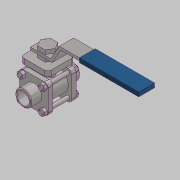
# Autodesk Inventor part: MANUAL BUTT WELD BALL VALVE DN15 304L
Saved by Autodesk Inventor 2017 (Build 210142000, 142)
## iProperties
Category: Plant Design Equipment
Company: Pocket Brewery Belgium
Created: 2017-11-25
Part Number: MANUAL BUTT WELD BALL VALVE DN15 304L
Material: 304L
Document SubType Name: Modeling
Designer: Demarec
Density: 8 g/cm^3
Appearance: Semi-Polished(1)
Description: BELVEN BV3
Author: Marc Crauwels
Title: Valves
Comments: This Valve is generated with the Pocket Brewery Valve App. This software is part of the Pocket Brewery Design Suite.
Autodesk Inventor part; units mm, degrees
ref_plane "YZ Plane" through (0, 0, 0) normal (1, 0, 0) x (0, 1, 0)
ref_plane "XZ Plane" through (0, 0, 0) normal (0, 1, 0) x (-1, 0, 0)
sketch "Sketch3" plane through (0, 0, 0) normal (0, 1, 0) x (-1, 0, 0)
  line L0 (-4.0756, 9.8393) -> (4.0756, 9.8393)
  line L1 (4.0756, 9.8393) -> (9.8393, 4.0756)
  line L2 (9.8393, 4.0756) -> (9.8393, -4.0756)
  line L3 (9.8393, -4.0756) -> (4.0756, -9.8393)
  line L4 (4.0756, -9.8393) -> (-4.0756, -9.8393)
  line L5 (-4.0756, -9.8393) -> (-9.8393, -4.0756)
  line L6 (-9.8393, -4.0756) -> (-9.8393, 4.0756)
  line L7 (-9.8393, 4.0756) -> (-4.0756, 9.8393)
  circle A0 centre (0, 0) radius 10.65
  line L8 (14.25, -19) -> (-14.25, -19)
  line L9 (-19, -14.25) -> (-19, 14.25)
  line L10 (-14.25, 19) -> (14.25, 19)
  line L11 (19, 14.25) -> (19, -14.25)
  line L12 (19, -19) -> (-19, 19) construction
  line L13 (-19, -19) -> (19, 19) construction
  circle A1 centre (0, 0) radius 9.8393
  arc A2 (19, 14.25) -> (14.25, 19) centre (14.25, 14.25) ccw
  arc A3 (-14.25, 19) -> (-19, 14.25) centre (-14.25, 14.25) ccw
  arc A4 (-19, -14.25) -> (-14.25, -19) centre (-14.25, -14.25) ccw
  arc A5 (14.25, -19) -> (19, -14.25) centre (14.25, -14.25) ccw
  circle A6 centre (0, 0) radius 8
  circle A7 centre (14.25, 14.25) radius 2.5
  circle A8 centre (0, 0) radius 14.65
  dimension "oSW" = 21.3
  dimension "oFlangeW" = 38
  dimension "d2" = 4.75
  dimension "oIntDia" = 16
  dimension "oMbolt" = 5
  dimension "d16" = 4
  constraints: 28 end point, 9 tangent, 8 centre point, 8 point on circle, 8 point on line, 5 coincident, 3 equal radius, 2 horizontal, 2 midpoint, 2 parallel, 2 perpendicular, 20 other
  measures "oFlangeW" distance of L12.start L13.start
  measures "d2" radius of A2
  measures "oIntDia" diameter of A6
  measures "oMbolt" diameter of A7
extrude "Extrusion1" add sketch "Sketch3" along normal mid plane 65 contours A0 L0 | L0 A1 L7 | L7 A0 | L0 L1 A1 | A1 | A1 L6 L7 | A0 L1 | L6 A0 | L1 L2 A1 | A1 L5 L6 | A0 L2 | L5 A0 | L2 L3 A1 | A1 L4 L5 | L4 A0 | A0 L3 | L3 L4 A1
extrude "Extrusion2" add sketch "Sketch3" along normal mid plane 37 contours A0 L0 | L7 A0 | A0 L1 | L6 A0 | A0 L2 | L5 A0 | L4 A0 | A0 L3 | L8 A4 L9 A3 L10 A2 L11 A5 | A7 | A8
extrude "Extrusion3" cut sketch "Sketch3" along normal mid plane 25 contours L8 A4 L9 A3 L10 A2 L11 A5 | A7
extrude "Extrusion4" add sketch "Sketch3" along normal mid plane 48 contours A7
sketch "Sketch4" plane through (0, -18.5, 0) normal (0, -1, 0) x (1, 0, 0)
  circle A0 centre (-14.25, 14.25) radius 2.5 projected
  line L0 (-12.0849, 10.5) -> (-16.4151, 10.5)
  line L1 (-16.4151, 10.5) -> (-18.5801, 14.25)
  line L2 (-18.5801, 14.25) -> (-16.4151, 18)
  line L3 (-16.4151, 18) -> (-12.0849, 18)
  line L4 (-12.0849, 18) -> (-9.9199, 14.25)
  line L5 (-9.9199, 14.25) -> (-12.0849, 10.5)
  point P0 (0, 0)
  dimension "d13" = 7.5
  constraints: 12 end point, 1 coincident, 1 horizontal, 13 other
  measures "d13" distance between parallel lines of L0 L3
extrude "Extrusion5" add sketch "Sketch4" along normal blind 4
mirror "Mirror1" about plane through (0, 0, 0) normal (0, 1, 0) of "Extrusion5"
pattern_circular "Circular Pattern1" count 4 over 360 about axis through (0, 0, 0) along (0, 1, 0) of "Extrusion5", "Extrusion4", "Mirror1"
ref_plane "Work Plane1" through (0, 0, 32) normal (0, 0, 1) x (1, 0, 0)
sketch "Sketch5" plane through (0, 0, 32) normal (0, 0, 1) x (1, 0, 0)
  line L0 (-13.25, -18) -> (13.25, -18)
  line L1 (18, -13.25) -> (18, 13.25)
  line L2 (13.25, 18) -> (-13.25, 18)
  line L3 (-18, 13.25) -> (-18, -13.25)
  line L4 (-18, -18) -> (18, 18) construction
  line L5 (18, -18) -> (-18, 18) construction
  arc A0 (-18, -13.25) -> (-13.25, -18) centre (-13.25, -13.25) ccw
  arc A1 (13.25, -18) -> (18, -13.25) centre (13.25, -13.25) ccw
  arc A2 (18, 13.25) -> (13.25, 18) centre (13.25, 13.25) ccw
  arc A3 (-13.25, 18) -> (-18, 13.25) centre (-13.25, 13.25) ccw
  point P0 (0, 0)
  dimension "d21" = 36
  dimension "d22" = 4.75
  constraints: 12 end point, 8 point on circle, 8 point on line, 8 tangent, 4 centre point, 3 equal radius, 2 midpoint, 2 parallel, 2 perpendicular, 1 horizontal
  measures "d21" distance of L4.start L5.start
  measures "d22" radius of A0
extrude "Extrusion6" add sketch "Sketch5" against normal blind 7
sketch "Sketch6" plane through (0, 0, 25) normal (0, 0, -1) x (-1, 0, 0)
  circle A0 centre (0, 0) radius 8
  dimension "d25" = 16
  constraints: 1 centre point, 1 coincident
  measures "d25" diameter of A0
extrude "Extrusion7" add sketch "Sketch6" along normal up to surface
sketch "Sketch8" plane through (0, 0, 32) normal (0, 0, 1) x (1, 0, 0)
  line L0 (-4.9075, -8.5) -> (-9.815, 0)
  line L1 (-9.815, 0) -> (-4.9075, 8.5)
  line L2 (-4.9075, 8.5) -> (4.9075, 8.5)
  line L3 (4.9075, 8.5) -> (9.815, 0)
  line L4 (9.815, 0) -> (4.9075, -8.5)
  line L5 (4.9075, -8.5) -> (-4.9075, -8.5)
  point P0 (0, 0)
  point P1 (0, 0)
  dimension "oSW2" = 17
  constraints: 12 end point, 1 coincident, 1 horizontal, 13 other
  measures "oSW2" distance between parallel lines of L2 L5
extrude "Extrusion8" add sketch "Sketch8" along normal blind 14
sketch "Sketch9" plane through (0, 0, 0) normal (0, 1, 0) x (-1, 0, 0)
  line L0 (-9.815, 32) -> (-9.815, 46) projected
  line L1 (-13.315, 37.25) -> (15.3357, 37.25)
  line L2 (15.3357, 37.25) -> (26.8827, 57.25)
  line L3 (26.8827, 57.25) -> (52.4, 57.25)
  line L4 (52.4, 57.25) -> (52.4, 60.75)
  line L5 (52.4, 60.75) -> (24.862, 60.75)
  line L6 (24.862, 60.75) -> (13.315, 40.75)
  line L7 (13.315, 40.75) -> (-13.315, 40.75)
  line L8 (-13.315, 40.75) -> (-13.315, 37.25)
  line L9 (-9.815, 39) -> (-13.315, 39) construction
  line L10 (17.4866, 40.9755) -> (14.4555, 42.7255) construction
  line L11 (52.4, 61.75) -> (131, 61.75)
  line L12 (131, 61.75) -> (131, 56.25)
  line L13 (131, 56.25) -> (52.4, 56.25)
  line L14 (52.4, 56.25) -> (52.4, 61.75)
  line L15 (9.815, 32) -> (9.815, 46) projected
  point P0 (0, 0)
  point P1 (52.4, 59)
  dimension "d32" = 60
  dimension "d33" = 3.5
  dimension "oHeightHandle" = 20
  dimension "d35" = 1
  dimension "d36" = 3.5
  dimension "d37" = 3.5
  dimension "oLenghtHandle" = 131
  dimension "d39" = 78.6
  constraints: 28 end point, 6 perpendicular, 4 midpoint, 4 parallel, 3 horizontal, 2 equal length, 2 point on line
  measures "d32" angle of L6 L7
  measures "d33" distance of L7.end L1.start
  measures "oHeightHandle" distance between parallel lines of L5 L7
  measures "d35" distance between parallel lines of L11 L5
  measures "d36" distance between parallel lines of L0 L8
  measures "d37" distance from line of L15 L6.end
  measures "oLenghtHandle" distance from line of point (0, 0) L12
  measures "d39" distance of L11.start L11.end
extrude "Extrusion9" add sketch "Sketch9" along normal mid plane 19 contours L1 L8 L7 L0 | L0 L7 L15 L1 | L15 L7 L6 L5 L4 L3 L2 L1
extrude "Extrusion10" add sketch "Sketch9" along normal mid plane 21 contours L4 L14 L11 L12 L13
chamfer "Chamfer1" distance 1 angle 45 2 edges at (10.65, 32.5, 0) (10.65, -32.5, 0)
equation "\"d2\" = 0.125 * oFlangeW"
equation "\"d13\" = 1.5 * oMbolt"
equation "\"d14\" = 0.8 * oMbolt"
equation "\"d22\" = d2"
equation "\"d25\" = oIntDia"
equation "\"d33\" = 0.25 * oHeightTop"
equation "\"d36\" = d33"
equation "\"d37\" = d36"
equation "\"d39\" = 0.6 * oLenghtHandle"
equation "\"oHeightTop\" = 14"
body "Solid1"
